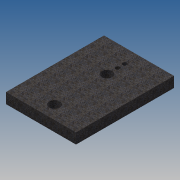
# Autodesk Inventor part: plinth
Saved by Autodesk Inventor 2014 SP1 (Build 180222100, 222)
## iProperties
Created: 2014-03-11
Part Number: plinth
Material: Concrete
Document SubType Name: Modeling
Designer: Dave
Density: 2.40731 g/cm^3
Appearance: Exposed Aggregate - Coarse
Mass: 77996.9 g
Surface Area: 17640 cm^2
Volume: 32400 cm^3
Author: Dave
Autodesk Inventor part; units mm, degrees
ref_plane "YZ Plane" through (0, 0, 0) normal (1, 0, 0) x (0, 1, 0)
ref_plane "XZ Plane" through (0, 0, 0) normal (0, 1, 0) x (-1, 0, 0)
ref_plane "XY Plane" through (0, 0, 0) normal (0, 0, 1) x (1, 0, 0)
sketch "Sketch1" plane through (0, 0, 0) normal (0, 1, 0) x (-1, 0, 0)
  line L0 (0, 0) -> (1000, 0)
  line L1 (1000, 0) -> (1000, 1400)
  line L2 (1000, 1400) -> (0, 1400)
  line L3 (0, 1400) -> (0, 0)
  dimension "d0" = 1000
  dimension "d1" = 1400
  constraints: 8 end point, 2 parallel, 1 horizontal, 1 perpendicular
  measures "d0" distance of L2.end L1.end
  measures "d1" distance of L2.end L0.start
extrude "base" add sketch "Sketch1" along normal blind 150
sketch "Sketch2" plane through (0, 150, 0) normal (0, 1, 0) x (1, 0, 0)
  circle A0 centre (-500, -457.2) radius 75
  line L0 (0, 0) -> (-1000, 0) projected
  line L1 (-1000, -1400) -> (0, -1400) projected
  line L2 (-500, 0) -> (-500, -1400) construction
  dimension "d4" = 150
  dimension "d38" = 457.2
  constraints: 2 end point, 2 midpoint, 1 centre point, 1 point on line
  measures "d4" diameter of A0
  measures "d38" distance from line of A0.centre L0
extrude "air" cut sketch "Sketch2" against normal through all
sketch "Sketch3" plane through (0, 150, 0) normal (0, 1, 0) x (1, 0, 0)
  circle A0 centre (-500, -457.2) radius 75 projected
  circle A1 centre (-500, -203.2) radius 30.48
  dimension "d7" = 60.96
  dimension "d8" = 254
  constraints: 1 centre point
  measures "d7" diameter of A1
  measures "d8" distance of A1.centre A0.centre
extrude "power" cut sketch "Sketch3" against normal blind 254 contours A1
sketch "Sketch4" plane through (0, 150, 0) normal (0, 1, 0) x (1, 0, 0)
  circle A0 centre (-500, -203.2) radius 30.48 projected
  circle A1 centre (-500, -457.2) radius 75 projected
  line L0 (0, -1400) -> (0, 0) projected
  circle A2 centre (-500, -304.8) radius 25.4
  line L1 (-500, -203.2) -> (-500, -457.2) construction
  dimension "d11" = 50.8
  dimension "d12" = 101.6
  constraints: 2 end point, 1 centre point, 1 parallel
  measures "d11" diameter of A2
  measures "d12" distance of A2.centre L1.start
hole "fibre" at (-500, 150, 304.8) direction (0, -1, 0) diameter 60.96 end through all
sketch "Sketch6" plane through (0, 150, 0) normal (0, 1, 0) x (1, 0, 0)
  circle A0 centre (-500, -457.2) radius 75 projected
  circle A1 centre (-500, -1207.2) radius 76.2
  dimension "d29" = 152.4
  dimension "d30" = 750
  constraints: 1 centre point
  measures "d29" diameter of A1
  measures "d30" distance of A1.centre A0.centre
hole "air2" at (-500, 150, 1207.2) direction (0, -1, 0) diameter 152.4 end through all
body "Solid1"
